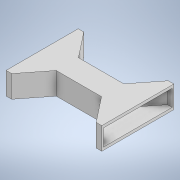
# Autodesk Inventor part: Metal_Shroud
Saved by Autodesk Inventor 2022 (Build 260153000, 153)
## iProperties
Created: 2022-01-23
Part Number: Metal_Shroud
Material: Generic
Document SubType Name: Modeling
Designer: Mlees
Density: 1 g/cm^3
Appearance: Default
Author: Mlees
Autodesk Inventor part; units mm, degrees
ref_plane "YZ Plane" through (0, 0, 0) normal (1, 0, 0) x (0, 1, 0)
ref_plane "XZ Plane" through (0, 0, 0) normal (0, 1, 0) x (-1, 0, 0)
ref_plane "XY Plane" through (0, 0, 0) normal (0, 0, 1) x (1, 0, 0)
sketch "Sketch1" plane through (0, 0, 0) normal (0, 1, 0) x (-1, 0, 0)
  line L0 (172.412, 0) -> (172.412, -65)
  line L1 (172.412, 0) -> (172.412, 65)
  line L2 (172.412, 65) -> (162.412, 65)
  line L3 (162.412, 65) -> (127.012, 20)
  line L4 (172.412, -65) -> (162.412, -65)
  line L5 (162.412, -65) -> (127.012, -20)
  line L6 (127.012, -20) -> (86.206, -20)
  line L7 (127.012, 20) -> (86.206, 20)
  line L8 (0, 0) -> (0, -65)
  line L9 (0, 0) -> (0, 65)
  line L10 (0, 65) -> (10, 65)
  line L11 (10, 65) -> (45.4, 20)
  line L12 (0, -65) -> (10, -65)
  line L13 (10, -65) -> (45.4, -20)
  line L14 (45.4, -20) -> (86.206, -20)
  line L15 (45.4, 20) -> (86.206, 20)
  dimension "d0" = 172.412
  dimension "d1" = 65
  dimension "d2" = 65
  dimension "d7" = 10
  constraints: 32 end point, 2 horizontal, 2 vertical
  measures "d0" distance of point (0, 0) L0.start
  measures "d1" distance of L0.start L0.end
  measures "d2" distance of L0.start L1.end
  measures "d7" distance of L1.end L2.end
extrude "Extrusion1" add sketch "Sketch1" along normal blind 5
sketch "Sketch2" plane through (0, 5, 0) normal (0, 1, 0) x (1, 0, 0)
  line L0 (-162.412, -65) -> (-127.012, -20) projected
  line L1 (-127.012, -20) -> (-162.412, -65)
  line L2 (-162.412, -65) -> (-172.412, -65)
  line L3 (-127.012, 20) -> (-162.412, 65) projected
  line L4 (-172.412, 65) -> (-162.412, 65)
  line L5 (-162.412, 65) -> (-127.012, 20)
  line L6 (-127.012, 20) -> (-45.4, 20)
  line L7 (-10, 65) -> (-45.4, 20) projected
  line L8 (-45.4, 20) -> (-10, 65)
  line L9 (-10, 65) -> (0, 65)
  line L10 (0, -65) -> (0, 65) projected
  line L11 (-45.4, -20) -> (-10, -65) projected
  line L12 (0, -65) -> (-10, -65)
  line L13 (-10, -65) -> (-45.4, -20)
  line L14 (-45.4, -20) -> (-127.012, -20)
  line L15 (-128.469, -17) -> (-163.869, -62)
  line L16 (-163.869, -62) -> (-169.412, -62)
  line L17 (-169.412, 62) -> (-163.869, 62)
  line L18 (-163.869, 62) -> (-128.469, 17)
  line L19 (-128.469, 17) -> (-43.943, 17)
  line L20 (-43.943, 17) -> (-8.543, 62)
  line L21 (-8.543, 62) -> (-3, 62)
  line L22 (-3, -62) -> (-8.543, -62)
  line L23 (-8.543, -62) -> (-43.943, -17)
  line L24 (-43.943, -17) -> (-128.469, -17)
  line L25 (-3, -62) -> (0, -62)
  line L26 (0, -65) -> (0, -62)
  line L27 (-3, 62) -> (0, 62)
  line L28 (0, 65) -> (0, 62)
  line L29 (-169.412, -62) -> (-172.412, -62)
  line L30 (-172.412, -65) -> (-172.412, -62)
  line L31 (-169.412, 62) -> (-172.412, 62)
  line L32 (-172.412, 62) -> (-172.412, 65)
  point P0 (0, 0)
  dimension "d10" = 3
  constraints: 56 end point, 6 parallel, 4 collinear, 3 perpendicular, 1 point on line, 1 vertical, 7 other
  measures "d10" distance between parallel lines of L14 L24
extrude "Extrusion2" add sketch "Sketch2" along normal blind 30
sketch "Sketch3" plane through (0, 35, 0) normal (0, 1, 0) x (1, 0, 0)
  line L0 (-172.412, 65) -> (-172.412, -65) projected
  line L1 (-172.412, -65) -> (-172.412, 65)
  line L2 (-162.412, 65) -> (-172.412, 65) projected
  line L3 (-172.412, 65) -> (-162.412, 65)
  line L4 (-45.4, 20) -> (-127.012, 20) projected
  line L5 (-162.412, 65) -> (-127.012, 20)
  line L6 (-127.012, 20) -> (-45.4, 20)
  line L7 (-45.4, 20) -> (-10, 65)
  line L8 (0, 65) -> (-10, 65) projected
  line L9 (-10, 65) -> (0, 65)
  line L10 (-10, -65) -> (0, -65) projected
  line L11 (0, 65) -> (0, -65)
  line L12 (0, -65) -> (-10, -65)
  line L13 (-127.012, -20) -> (-45.4, -20) projected
  line L14 (-10, -65) -> (-45.4, -20)
  line L15 (-45.4, -20) -> (-127.012, -20)
  line L16 (-162.412, -65) -> (-127.012, -20) projected
  line L17 (-127.012, -20) -> (-162.412, -65)
  line L18 (-172.412, -65) -> (-162.412, -65) projected
  line L19 (-162.412, -65) -> (-172.412, -65)
  point P0 (0, 0)
  constraints: 24 end point, 6 collinear, 2 parallel, 1 perpendicular, 1 vertical
extrude "Extrusion3" add sketch "Sketch3" along normal blind 5
body "Solid1"
